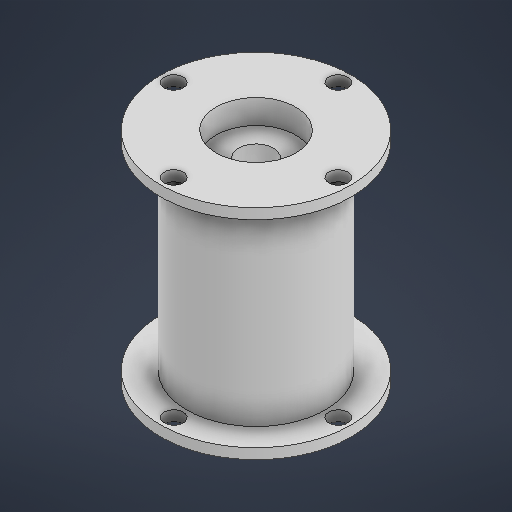
# Autodesk Inventor part: cabezal extrusora
Saved by Autodesk Inventor 2026.1 (Build 301233020, 233B)
## iProperties
Created: 2025-12-04
Part Number: cabezal extrusora
Material: Genérico
Document SubType Name: Modeling
Designer: benja
Density: 1 g/cm^3
Appearance: Valor por defecto
Author: benja
Autodesk Inventor part; units mm, degrees
ref_plane "YZ Plane" through (0, 0, 0) normal (1, 0, 0) x (0, 1, 0)
ref_plane "XZ Plane" through (0, 0, 0) normal (0, 1, 0) x (-1, 0, 0)
ref_plane "XY Plane" through (0, 0, 0) normal (0, 0, 1) x (1, 0, 0)
sketch "Boceto1" plane through (0, 0, 0) normal (0, 1, 0) x (-1, 0, 0)
  circle A0 centre (0, 0) radius 20
  dimension "d0" = 40
  constraints: 1 centre point, 1 coincident
  measures "d0" diameter of A0
extrude "Extrusión1" add sketch "Boceto1" along normal blind 60
sketch "Boceto10" plane through (0, 0, 0) normal (0, -1, 0) x (1, 0, 0)
  circle A0 centre (0, 0) radius 11
  dimension "d34" = 22
  constraints: 1 centre point, 1 coincident
  measures "d34" diameter of A0
extrude "Extrusión2" cut sketch "Boceto10" against normal blind 35
sketch "Boceto11" plane through (0, 0, 0) normal (1, 0, 0) x (0, 1, 0)
  line L0 (35, -11) -> (35, 11) projected
  line L1 (35, 0) -> (35, 11)
  line L2 (35, 0) -> (45, 0)
  line L3 (45, 0) -> (45, 5)
  line L4 (45, 5) -> (35, 11)
  point P0 (0, 0)
  dimension "d37" = 10
  dimension "d38" = 5
  constraints: 8 end point, 2 perpendicular, 1 collinear, 1 midpoint
  measures "d37" distance of L1.start L2.end
  measures "d38" distance of L2.end L3.end
revolve "Revolución6" cut sketch "Boceto11" angle 360 about axis through (0, 35, 0) along (0, -1, 0)
sketch "Boceto12" plane through (0, 45, 0) normal (0, -1, 0) x (1, 0, 0)
  circle A0 centre (0, 0) radius 5
  constraints: 1 centre point, 1 coincident
extrude "Extrusión3" cut sketch "Boceto12" against normal blind 35
sketch "Boceto13" plane through (0, 60, 0) normal (0, 1, 0) x (1, 0, 0)
  circle A0 centre (0, 0) radius 5 projected
  circle A1 centre (0, 0) radius 20
  dimension "d42" = 40
  constraints: 1 centre point, 1 coincident
  measures "d42" diameter of A1
extrude "Extrusión4" cut sketch "Boceto13" against normal blind 1
sketch "Boceto14" plane through (0, 60, 0) normal (0, 1, 0) x (1, 0, 0)
  circle A0 centre (0, 0) radius 27.5
  dimension "d45" = 55
  constraints: 1 centre point, 1 coincident
  measures "d45" diameter of A0
extrude "Extrusión5" add sketch "Boceto14" against normal blind 3
sketch "Boceto15" plane through (0, 57, 0) normal (0, -1, 0) x (1, 0, 0)
  circle A0 centre (0, 0) radius 11 projected
  circle A1 centre (0, 0) radius 5
  constraints: 1 centre point, 1 coincident
extrude "Extrusión6" cut sketch "Boceto15" against normal blind 10 contours A1
sketch "Boceto16" plane through (0, 0, 0) normal (0, -1, 0) x (1, 0, 0)
  circle A0 centre (0, 0) radius 27.5
  circle A1 centre (0, 0) radius 17.05
  dimension "d50" = 34.1
  constraints: 2 centre point, 2 coincident
  measures "d50" diameter of A1
extrude "Extrusión7" add sketch "Boceto16" along normal blind 3
sketch "Boceto17" plane through (0, 60, 0) normal (0, 1, 0) x (1, 0, 0)
  circle A0 centre (0, 0) radius 20
  circle A1 centre (0, 0) radius 27.5
  circle A2 centre (0, -23.75) radius 2.75
  circle A3 centre (-23.75, 0) radius 2.75
  circle A4 centre (0, 23.75) radius 2.75
  circle A5 centre (23.75, 0) radius 2.75
  dimension "d53" = 40
  dimension "d58" = 5.5
  dimension "d59" = 5.5
  dimension "d60" = 5.5
  dimension "d61" = 5.5
  constraints: 6 centre point, 2 coincident
  measures "d53" diameter of A0
  measures "d58" diameter of A2
  measures "d59" diameter of A3
  measures "d60" diameter of A4
  measures "d61" diameter of A5
extrude "Extrusión8" cut sketch "Boceto17" against normal blind 100 contours A2 | A3 | A4 | A5
sketch "Boceto18" plane through (0, 60, 0) normal (0, 1, 0) x (1, 0, 0)
  circle A0 centre (0, 0) radius 11.5
  dimension "d64" = 23
  constraints: 1 centre point, 1 coincident
  measures "d64" diameter of A0
extrude "Extrusión9" cut sketch "Boceto18" against normal blind 7
